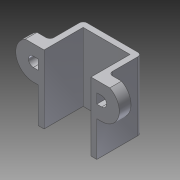
# Autodesk Inventor part: fixation moteur
Saved by Autodesk Inventor 2014 SP2 (Build 180246200, 246)
## iProperties
Created: 2015-03-17
Part Number: fixation moteur
Material: Plastique ABS
Document SubType Name: Modeling
Designer: sd
Density: 1.06 g/cm^3
Appearance: Lisse - Blanc
Mass: 1.19861 g
Surface Area: 16.0973 cm^2
Volume: 1.13077 cm^3
Author: sd
Autodesk Inventor part; units mm, degrees
ref_plane "YZ Plane" through (0, 0, 0) normal (1, 0, 0) x (0, 1, 0)
ref_plane "XZ Plane" through (0, 0, 0) normal (0, 1, 0) x (-1, 0, 0)
ref_plane "XY Plane" through (0, 0, 0) normal (0, 0, 1) x (1, 0, 0)
sketch "Esquisse1" plane through (0, 0, 0) normal (0, 0, 1) x (1, 0, 0)
  line L0 (7.5, 0) -> (-7.5, 0)
  line L1 (-7.5, 0) -> (-7.5, 11.5)
  line L2 (-7.5, 11.5) -> (7.5, 11.5)
  line L3 (7.5, 11.5) -> (7.5, 0)
  point P0 (0, 0)
  dimension "d0" = 15
  dimension "d1" = 11.5
  dimension "d2" = 0
  dimension "d3" = 7.5
  constraints: 8 end point, 2 parallel, 1 horizontal, 1 perpendicular
  measures "d0" distance of L1.end L2.end
  measures "d1" distance of L0.end L1.end
  measures "d2" vertical distance of L0.end point (0, 0)
  measures "d3" horizontal distance of point (0, 0) L1.end
extrude "Extrusion1" add sketch "Esquisse1" along normal blind 17.5
sketch "Esquisse2" plane through (0, 0, 17.5) normal (0, 0, 1) x (1, 0, 0)
  line L0 (-7.5, 0) -> (7.5, 0) projected
  line L1 (7.5, 0) -> (7.5, 11.5) projected
  line L2 (7.5, 11.5) -> (-7.5, 11.5) projected
  line L3 (-7.5, 11.5) -> (-7.5, 0) projected
  line L4 (-6, 0) -> (6, 0)
  line L5 (6, 0) -> (6, 10)
  line L6 (6, 10) -> (-6, 10)
  line L7 (-6, 10) -> (-6, 0)
  point P0 (0, 0)
  dimension "d6" = 1.5
  dimension "d7" = 1.5
  dimension "d8" = 1.5
  constraints: 8 end point, 2 parallel, 1 horizontal, 1 perpendicular, 1 point on line
  measures "d6" distance between parallel lines of L2 L6
  measures "d7" distance between parallel lines of L7 L3
  measures "d8" distance between parallel lines of L1 L5
extrude "Extrusion2" cut sketch "Esquisse2" against normal through all contours L7 L6 L5 L0
fillet "Congé1" radius 1 2 edges at (7.5, 11.5, 8.75) (-7.5, 11.5, 8.75)
sketch "Esquisse4" plane through (7.5, 0, 0) normal (0, -1, 0) x (1, 0, 0)
  line L0 (0, 0) -> (0, 17.5) projected
  circle A0 centre (-16.25, 13.5) radius 1.25
  circle A1 centre (1.25, 13.5) radius 1.25
  line L1 (1.25, 9) -> (0, 9)
  line L2 (-16.25, 9) -> (-15, 9)
  line L3 (-16.25, 14.75) -> (-15, 14.75)
  line L4 (-16.25, 12.25) -> (-15, 12.25)
  line L5 (1.25, 14.75) -> (0, 14.75)
  line L6 (1.25, 12.25) -> (0, 12.25)
  line L7 (0, 12.25) -> (0, 9)
  line L8 (0, 17.5) -> (0, 14.75)
  line L9 (-15, 17.5) -> (-15, 14.75)
  line L10 (-15, 12.25) -> (-15, 9)
  arc A2 (-18.3116, 17.5) -> (-16.25, 9) centre (-16.25, 13.5) ccw
  line L11 (-13.5, 17.5) -> (-1.5, 17.5) projected
  arc A3 (1.25, 9) -> (3.3116, 17.5) centre (1.25, 13.5) ccw
  line L12 (-18.3116, 17.5) -> (-15, 17.5)
  line L13 (0, 17.5) -> (3.3116, 17.5)
  point P0 (-7.5, 0)
  dimension "d12" = 2.5
  dimension "d13" = 2.5
  dimension "d14" = 17.5
  dimension "d15" = 8.75
  dimension "d18" = 4
  dimension "d22" = 4.5
  dimension "d23" = 3.25
  dimension "d24" = 5.25
  dimension "d25" = 4.5
  dimension "d26" = 3.25
  dimension "d27" = 152.734
  dimension "d28" = 152.734
  constraints: 24 end point, 8 point on circle, 6 tangent, 4 centre point, 4 collinear, 3 parallel, 3 perpendicular, 3 point on line
  measures "d12" diameter of A0
  measures "d13" diameter of A1
  measures "d14" distance of A1.centre A0.centre
  measures "d15" horizontal distance of point (-7.5, 0) A0.centre
  measures "d18" vertical distance of L0.end A1.centre
  measures "d22" radius of A2
  measures "d23" distance of L4.end L2.end
  measures "d24" distance from line of L11 L4.end
  measures "d25" radius of A3
  measures "d26" distance between parallel lines of L6 L1
extrude "Extrusion5" add sketch "Esquisse4" against normal blind 3 contours L0 L6 A1 L5 L13 A3 L1 | A0 L4 L10 L2 A2 L12 L9 L3
fillet "Congé2" radius 1 4 edges at (-7.5, 3, 10.625) (-7.5, 3, 16.125) (7.5, 3, 16.125) (7.5, 3, 10.625)
equation "\"d3\" = 0.5 * d0"
equation "\"d15\" = 0.5 * d14"
